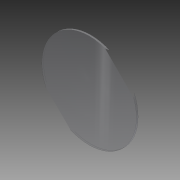
# Autodesk Inventor part: Build_170mm_Borosilicate
Saved by Autodesk Inventor 2014 (Build 180170000, 170)
## iProperties
Created: 2014-02-12
Part Number: Build_170mm_Borosilicate
Material: Glass
Document SubType Name: Modeling
Designer: ThatOtherGuy
Density: 2.42 g/cm^3
Mass: 164.788 g
Surface Area: 469.982 cm^2
Volume: 68.094 cm^3
Appearance: Clear
Author: ThatOtherGuy
Autodesk Inventor part; units mm, degrees
ref_plane "YZ Plane" through (0, 0, 0) normal (1, 0, 0) x (0, 1, 0)
ref_plane "XZ Plane" through (0, 0, 0) normal (0, 1, 0) x (-1, 0, 0)
ref_plane "XY Plane" through (0, 0, 0) normal (0, 0, 1) x (1, 0, 0)
sketch "Sketch1" plane through (0, 0, 0) normal (0, 1, 0) x (-1, 0, 0)
  circle A0 centre (0, 0) radius 85
  circle A1 centre (0, 0) radius 110
  dimension "d0" = 170
  dimension "d6" = 220
  constraints: 2 centre point, 2 coincident
  measures "d0" diameter of A0
  measures "d6" diameter of A1
extrude "Extrusion1" add sketch "Sketch1" along normal blind 3 contours A0
body "Solid1"
